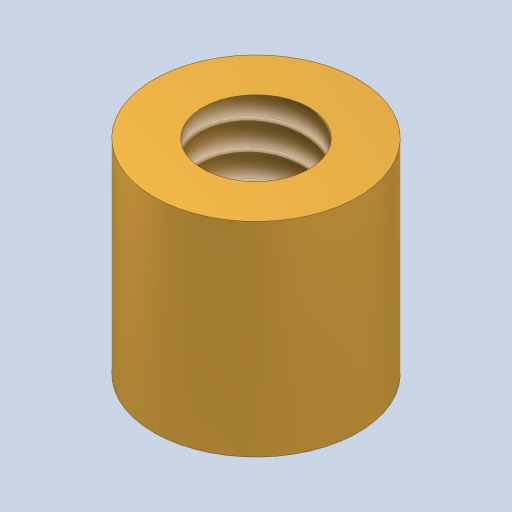
# Autodesk Inventor part: FB-2001
Saved by Autodesk Inventor 2023 (Build 270158000, 158)
## iProperties
Created: 2024-11-11
Part Number: FB-2001
Material: Generic
Document SubType Name: Modeling
Designer: kiyo
Density: 1 g/cm^3
Appearance: 真鍮 - サテン
Mass: 0.0334658 g
Surface Area: 0.878976 cm^2
Volume: 0.0334658 cm^3
Author: kiyo
Autodesk Inventor part; units mm, degrees
ref_plane "YZ Plane" through (0, 0, 0) normal (1, 0, 0) x (0, 1, 0)
ref_plane "XZ Plane" through (0, 0, 0) normal (0, 1, 0) x (-1, 0, 0)
ref_plane "XY Plane" through (0, 0, 0) normal (0, 0, 1) x (1, 0, 0)
sketch "スケッチ1" plane through (0, 0, 0) normal (0, 0, 1) x (1, 0, 0)
  circle A0 centre (0, 0) radius 1.5
  dimension "d0" = 3
  constraints: 2 coincident, 1 centre point
  measures "d0" diameter of A0
extrude "押し出し1" add sketch "スケッチ1" along normal blind 3
hole "穴1" at (0, 0, 0) direction (0, 0, 1) diameter 1.567 depth 6.3 tip angle 118 thread size "M2x0.4" designation "M2" class "6H" standard "GB Metric profile"
